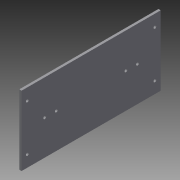
# Autodesk Inventor part: 000201
Saved by Autodesk Inventor 2015 (Build 190159000, 159)
## iProperties
Created: 2015-05-27
Part Number: 000201
Material: Generic
Document SubType Name: Modeling
Designer: Wesley
Density: 1 g/cm^3
Appearance: Default
Author: Wesley
Autodesk Inventor part; units mm, degrees
ref_plane "YZ Plane" through (0, 0, 0) normal (1, 0, 0) x (0, 1, 0)
ref_plane "XZ Plane" through (0, 0, 0) normal (0, 1, 0) x (-1, 0, 0)
ref_plane "XY Plane" through (0, 0, 0) normal (0, 0, 1) x (1, 0, 0)
sketch "Sketch1" plane through (0, 0, 0) normal (1, 0, 0) x (0, 1, 0)
  line L0 (0, 0) -> (76.2, 0)
  line L1 (76.2, 0) -> (76.2, -152.4)
  line L2 (76.2, -152.4) -> (0, -152.4)
  line L3 (0, -152.4) -> (0, 0)
  dimension "d0" = 76.2
  dimension "d1" = 152.4
  constraints: 8 end point, 2 parallel, 1 horizontal, 1 perpendicular
  measures "d0" distance of L0.start L0.end
  measures "d1" distance of L2.end L0.start
extrude "Extrusion1" add sketch "Sketch1" along normal blind 2.54
sketch "Sketch2" plane through (2.54, 0, 0) normal (1, 0, 0) x (0, 0, -1)
  line L0 (0, 76.2) -> (0, 0) projected
  line L1 (0, 0) -> (152.4, 0) projected
  line L2 (152.4, 0) -> (152.4, 76.2) projected
  line L3 (152.4, 76.2) -> (0, 76.2) projected
  line L4 (6.35, 69.85) -> (6.35, 6.35) construction
  line L5 (6.35, 6.35) -> (146.05, 6.35) construction
  line L6 (146.05, 6.35) -> (146.05, 69.85) construction
  line L7 (146.05, 69.85) -> (6.35, 69.85) construction
  point P0 (6.35, 63.5)
  point P1 (6.35, 12.7)
  point P2 (146.05, 12.7)
  point P3 (146.05, 63.5)
  dimension "d4" = 6.35
  dimension "d5" = 12.7
  dimension "d6" = 12.7
  dimension "d7" = 12.7
  dimension "d8" = 12.7
  constraints: 8 end point, 4 point on line, 3 other
  measures "d4" distance between parallel lines of L3 L7
  measures "d5" distance from line of L3 point (6.35, 63.5)
  measures "d6" distance from line of L1 point (6.35, 12.7)
  measures "d7" distance from line of point (146.05, 12.7) L1
  measures "d8" distance from line of L3 point (146.05, 63.5)
hole "Hole1" at (2.54, 63.5, -6.35) at (2.54, 12.7, -6.35) at (2.54, 12.7, -146.05) at (2.54, 63.5, -146.05) direction (-1, 0, 0) diameter 3.175 depth 25.4 tip angle 118
sketch "Sketch3" plane through (2.54, 0, 0) normal (1, 0, 0) x (0, 0, -1)
  circle A0 centre (146.05, 12.7) radius 1.5875 projected
  circle A1 centre (6.35, 63.5) radius 1.5875 projected
  circle A2 centre (6.35, 12.7) radius 1.5875 projected
  circle A3 centre (146.05, 63.5) radius 1.5875 projected
  line L0 (0, 76.2) -> (0, 0) construction
  line L1 (0, 0) -> (152.4, 0) construction
  line L2 (152.4, 0) -> (152.4, 76.2) construction
  line L3 (152.4, 76.2) -> (0, 76.2) construction
  line L4 (-29.9282, 38.1) -> (171.8832, 38.1) construction
  point P0 (38.1, 38.1)
  point P1 (127, 38.1)
  point P2 (114.3, 38.1)
  point P3 (25.4, 38.1)
  dimension "d16" = 38.1
  dimension "d17" = 25.4
  dimension "d18" = 12.7
  dimension "d19" = 12.7
  dimension "d20" = 25.4
  constraints: 4 point on line, 2 end point, 1 horizontal
  measures "d16" distance between parallel lines of L1 L4
  measures "d17" distance from line of L0 point (25.4, 38.1)
  measures "d18" distance of point (25.4, 38.1) point (38.1, 38.1)
  measures "d19" distance of point (127, 38.1) point (114.3, 38.1)
  measures "d20" distance from line of L2 point (127, 38.1)
hole "Hole2" at (2.54, 38.1, -38.1) at (2.54, 38.1, -127) at (2.54, 38.1, -114.3) at (2.54, 38.1, -25.4) direction (-1, 0, 0) diameter 3.175 depth 25.4 tip angle 118
body "Solid1"
